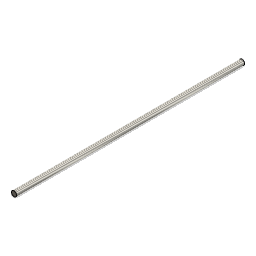
8mm T8 Lead Screw (345mm) v1 (Autodesk Fusion 360 design; units mm, degrees)
Autodesk Fusion 360 part; units mm, degrees
sketch "Sketch1" plane through (0, 0, 0) normal (0, 0, 1) x (1, 0, 0)
  circle A0 centre (0, 0) radius 4
  dimension "d1" = 8
  constraint coincident A0.centre origin
  measures "d1" diameter of A0
extrude "Extrude1" add sketch "Sketch1" along normal blind 345
thread "Thread1" "ISO Metric Trapezoidal Threads 8.0 TR8x1.5 7e" major diameter 7.925 minor diameter 6.0605 pitch 1.5 angle 30 resizes the face on face at (-1.5959, -3.6679, 230)
